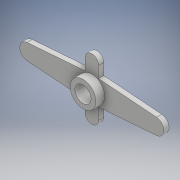
# Autodesk Inventor part: orczyk_k
Saved by Autodesk Inventor 2018 (Build 220112000, 112)
## iProperties
Created: 2020-10-02
Part Number: orczyk_k
Material: Ogólny
Document SubType Name: Modeling
Designer: Raven
Density: 1 g/cm^3
Appearance: Domyślna
Author: Raven
Autodesk Inventor part; units mm, degrees
ref_plane "YZ Plane" through (0, 0, 0) normal (1, 0, 0) x (0, 1, 0)
ref_plane "XZ Plane" through (0, 0, 0) normal (0, 1, 0) x (-1, 0, 0)
ref_plane "XY Plane" through (0, 0, 0) normal (0, 0, 1) x (1, 0, 0)
sketch "Szkic1" plane through (0, 0, 0) normal (0, 1, 0) x (-1, 0, 0)
  line L0 (0, 0) -> (19.6, 0) construction
  line L1 (0, 0) -> (-19.6, 0) construction
  line L2 (0, 0) -> (0, 8.3) construction
  line L3 (0, 0) -> (0, -8.3) construction
  circle A0 centre (0, 0) radius 2.2 construction
  line L4 (0, -8.3) -> (0, -6.45) construction
  circle A1 centre (0, -6.45) radius 1.85 construction
  line L5 (0, 8.3) -> (0, 6.45) construction
  circle A2 centre (0, 6.45) radius 1.85 construction
  circle A3 centre (0, 0) radius 3.5 construction
  line L6 (19.6, 0) -> (17.45, 0) construction
  circle A4 centre (17.45, 0) radius 2.15 construction
  line L7 (-19.6, 0) -> (-17.45, 0) construction
  circle A5 centre (-17.45, 0) radius 2.15 construction
  line L8 (0, 3.5) -> (-17.6151, 2.1437) construction
  line L9 (0, -3.5) -> (-17.6151, -2.1437) construction
  line L10 (0, 3.5) -> (17.6151, 2.1437) construction
  line L11 (0, -3.5) -> (17.6151, -2.1437) construction
  arc A6 (1.85, 6.45) -> (-1.85, 6.45) centre (0, 6.45) ccw
  arc A7 (-1.85, -6.45) -> (1.85, -6.45) centre (0, -6.45) ccw
  arc A8 (17.6151, -2.1437) -> (17.6151, 2.1437) centre (17.45, 0) ccw
  arc A9 (-17.6151, 2.1437) -> (-17.6151, -2.1437) centre (-17.45, 0) ccw
  circle A10 centre (0, 0) radius 2.2
  line L12 (1.85, 6.45) -> (1.85, -6.45) construction
  line L13 (-1.85, 6.45) -> (-1.85, -6.45) construction
  line L14 (1.85, 3.3576) -> (1.85, 6.45)
  line L15 (-1.85, 3.3576) -> (-1.85, 6.45)
  line L16 (-1.85, -3.3576) -> (-1.85, -6.45)
  line L17 (1.85, -3.3576) -> (1.85, -6.45)
  line L18 (1.85, -3.3576) -> (17.6151, -2.1437)
  line L19 (1.85, 3.3576) -> (17.6151, 2.1437)
  line L20 (-1.85, 3.3576) -> (-17.6151, 2.1437)
  line L21 (-1.85, -3.3576) -> (-17.6151, -2.1437)
  dimension "d0" = 19.6
  dimension "d1" = 19.6
  dimension "d2" = 8.3
  dimension "d3" = 8.3
  dimension "d4" = 4.4
  dimension "d5" = 1.85
  dimension "d6" = 1.85
  dimension "d7" = 7
  dimension "d8" = 2.15
  dimension "d9" = 2.15
  constraints: 44 end point, 26 point on circle, 14 point on line, 11 centre point, 8 tangent, 7 coincident, 7 parallel, 4 collinear, 2 horizontal, 2 vertical, 1 concentric
  measures "d0" distance of L0.start L0.end
  measures "d1" distance of L0.start L1.end
  measures "d2" distance of L0.start L2.end
  measures "d3" distance of L0.start L3.end
  measures "d4" diameter of A0
  measures "d5" distance of L3.end L4.end
  measures "d6" distance of L2.end L5.end
  measures "d7" diameter of A3
  measures "d8" distance of L0.end L6.end
  measures "d9" distance of L1.end L7.end
extrude "Wyciągnięcie proste1" add sketch "Szkic1" along normal blind 1.4
sketch "Szkic2" plane through (0, 0, 0) normal (0, -1, 0) x (1, 0, 0)
  circle A0 centre (0, 0) radius 2.2 projected
  circle A1 centre (0, 0) radius 3.5
  dimension "d12" = 7
  constraints: 1 centre point, 1 coincident
  measures "d12" diameter of A1
extrude "Wyciągnięcie proste2" add sketch "Szkic2" along normal blind 2.4
